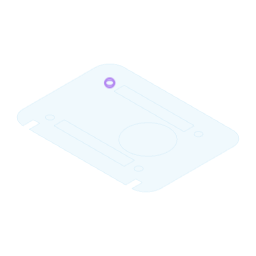
Seeed MT3620 Mini Dev Case (Autodesk Fusion 360 design; units mm, degrees)
Autodesk Fusion 360 part; units mm, degrees
sketch "Sketch1" plane through (0, 0, 0) normal (0, 1, 0) x (1, 0, 0)
  circle A0 centre (8.5, -10) radius 1.575
  circle A1 centre (51.5, -10) radius 1.575
  circle A2 centre (8.5, -39) radius 1.575
  circle A3 centre (51.5, -39) radius 1.575
  line L0 (5.5, 0) -> (58.2, 0)
  line L1 (65.2, -7) -> (65.2, -42)
  line L2 (58.2, -49) -> (5.5, -49)
  line L3 (-1.5, -42) -> (-1.5, -7)
  arc A4 (5.5, 0) -> (-1.5, -7) centre (5.5, -7) ccw
  arc A5 (65.2, -7) -> (58.2, 0) centre (58.2, -7) ccw
  arc A6 (-1.5, -42) -> (5.5, -49) centre (5.5, -42) ccw
  arc A7 (58.2, -49) -> (65.2, -42) centre (58.2, -42) ccw
  circle A8 centre (9, -34) radius 1
  line L4 (29.5, -28.775) -> (32, -28.775) construction
  line L5 (32, -28.775) -> (32, -35.275) construction
  line L6 (32, -35.275) -> (29.5, -35.275) construction
  line L7 (29.5, -35.275) -> (29.5, -28.775) construction
  circle A9 centre (8.5, -39) radius 2.075 construction
  circle A10 centre (8.5, -10) radius 2.075 construction
  circle A11 centre (51.5, -10) radius 2.075 construction
  circle A12 centre (51.5, -39) radius 2.075 construction
  line L8 (33, -27.775) -> (33, -36.275)
  line L9 (33, -36.275) -> (28.5, -36.275)
  line L10 (28.5, -36.275) -> (28.5, -27.775)
  line L11 (28.5, -27.775) -> (33, -27.775)
  line L12 (12.8, -11.5462) -> (11.2, -11.5462) construction
  line L13 (11.2, -11.5462) -> (11.2, -13.4538) construction
  line L14 (11.2, -13.4538) -> (12.8, -13.4538) construction
  line L15 (12.8, -13.4538) -> (12.8, -11.5462) construction
  line L16 (12.8, -11.5462) -> (11.2, -13.4538) construction
  line L17 (11.2, -11.5462) -> (12.8, -13.4538) construction
  line L18 (12.8, -9.2336) -> (11.2, -9.2336) construction
  line L19 (11.2, -9.2336) -> (11.2, -10.7664) construction
  line L20 (11.2, -10.7664) -> (12.8, -10.7664) construction
  line L21 (12.8, -10.7664) -> (12.8, -9.2336) construction
  line L22 (12.8, -9.2336) -> (11.2, -10.7664) construction
  line L23 (11.2, -9.2336) -> (12.8, -10.7664) construction
  line L24 (11.2, -9.2336) -> (11.2, -13.4538)
  line L25 (11.2, -13.4538) -> (12.8, -13.4538)
  line L26 (12.8, -13.4538) -> (12.8, -9.2336)
  line L27 (12.8, -9.2336) -> (11.2, -9.2336)
  line L28 (8.5, -39) -> (51.5, -39) construction
  line L29 (51.5, -39) -> (51.5, -10) construction
  line L30 (51.5, -10) -> (8.5, -10) construction
  line L31 (8.5, -10) -> (8.5, -39) construction
  line L32 (14.3, -14.9538) -> (14.3, -7.7336)
  line L33 (14.3, -7.7336) -> (9.7, -7.7336)
  line L34 (9.7, -7.7336) -> (9.7, -14.9538)
  line L35 (9.7, -14.9538) -> (14.3, -14.9538)
  point P0 (12, -10)
  point P1 (12, -12.5)
  point P2 (12, -12.5)
  point P3 (12, -10)
  dimension "d1" = 3.15
  dimension "d2" = 3.15
  dimension "d3" = 3.15
  dimension "d4" = 3.15
  dimension "d13" = 7
  dimension "d14" = 7
  dimension "d15" = 7
  dimension "d16" = 7
  dimension "d17" = 2
  dimension "d18" = 5
  dimension "d19" = 0.5
  dimension "d21" = 23.5
  dimension "d22" = 2.5
  dimension "d23" = 6.5
  dimension "d24" = 4.15
  dimension "d25" = 4.15
  dimension "d26" = 4.15
  dimension "d27" = 4.15
  dimension "d29" = -1
  dimension "d30" = 3.5
  dimension "d39" = 29
  dimension "d40" = 29
  dimension "d41" = 10
  dimension "d42" = 10
  dimension "d50" = 43
  dimension "d88" = 1.5
  constraint horizontal L0
  constraint vertical L1
  constraint horizontal L2
  constraint vertical L3
  constraint tangent L3 A4
  constraint tangent L0 A4
  constraint tangent L0 A5
  constraint tangent L1 A5
  constraint tangent L3 A6
  constraint tangent L2 A6
  constraint tangent L2 A7
  constraint tangent L1 A7
  constraint horizontal L4
  constraint vertical L5
  constraint horizontal L6
  constraint vertical L7
  constraint concentric A2 A9
  constraint concentric A0 A10
  constraint concentric A1 A11
  constraint concentric A3 A12
  constraint horizontal L12
  constraint perpendicular L12 L13
  constraint parallel L12 L14
  constraint parallel L13 L15
  constraint coincident L16 P2
  constraint coincident L17 P2
  constraint coincident P2 P1
  constraint horizontal L18
  constraint perpendicular L18 L19
  constraint parallel L18 L20
  constraint parallel L19 L21
  constraint coincident L22 P3
  constraint coincident L23 P3
  constraint coincident P3 P0
  constraint perpendicular L14 L24
  constraint perpendicular L18 L26
  constraint horizontal L28
  constraint vertical L29
  constraint horizontal L30
  constraint vertical L31
  constraint coincident A1.centre A11.centre
  constraint coincident A2.centre A9.centre
  measures "d1" diameter of A0
  measures "d2" diameter of A1
  measures "d3" diameter of A2
  measures "d4" diameter of A3
  measures "d13" radius of A4
  measures "d14" radius of A5
  measures "d15" radius of A6
  measures "d16" radius of A7
  measures "d17" diameter of A8
  measures "d18" vertical distance of A2.centre A8.centre
  measures "d19" horizontal distance of A2.centre A8.centre
  measures "d21" distance of A2.centre L5
  measures "d22" distance of L4.start L4.end
  measures "d23" distance of L4.start L6.end
  measures "d24" diameter of A9
  measures "d25" diameter of A10
  measures "d26" diameter of A11
  measures "d27" diameter of A12
  measures "d30" distance of A0.centre P3
  measures "d39" distance of A1.centre A3.centre
  measures "d40" distance of A0.centre A2.centre
  measures "d41" distance of L2 L28
  measures "d42" distance of L0 L30
  measures "d50" distance of A0.centre A1.centre
extrude "Extrude1" add sketch "Sketch1" along normal blind 3 contours L0 L1 L2 L3 A4 A5 A6 A7 makes body 1
ref_plane "WorkPlane1" through (31.85, -10.5, 24.5) normal (0, -1, 0) x (-1, 0, 0)
sketch "Sketch2" plane through (31.85, -10.5, 21.35) normal (0, -1, 0) x (1, 0, 0)
  line L0 (-33.35, 20.65) -> (-33.35, -14.35)
  arc A0 (-26.35, 27.65) -> (-33.35, 20.65) centre (-26.35, 20.65) ccw
  line L1 (26.35, 27.65) -> (-26.35, 27.65)
  arc A1 (33.35, 20.65) -> (26.35, 27.65) centre (26.35, 20.65) ccw
  line L2 (33.35, -14.35) -> (33.35, 20.65)
  arc A2 (26.35, -21.35) -> (33.35, -14.35) centre (26.35, -14.35) ccw
  line L3 (-26.35, -21.35) -> (26.35, -21.35)
  arc A3 (-33.35, -14.35) -> (-26.35, -21.35) centre (-26.35, -14.35) ccw
  circle A4 centre (-23.35, 17.65) radius 1.575
  circle A5 centre (19.65, 17.65) radius 1.575
  circle A6 centre (19.65, -11.35) radius 1.575
  line L4 (19.65, 17.65) -> (19.65, 3.15) construction
  line L5 (19.65, 17.65) -> (19.65, -11.35) construction
  circle A7 centre (9.65, 3.15) radius 10
  line L6 (15.15, 20.15) -> (-18.85, 20.15)
  line L7 (-18.85, 20.15) -> (-18.85, 15.15)
  line L8 (-18.85, 15.15) -> (15.15, 15.15)
  line L9 (15.15, 15.15) -> (15.15, 20.15)
  line L10 (15.15, 20.15) -> (-18.85, 15.15) construction
  line L11 (-18.85, 20.15) -> (15.15, 15.15) construction
  line L12 (-23.35, 17.65) -> (19.65, 17.65) construction
  line L13 (-23.35, -11.35) -> (19.65, -11.35) construction
  line L14 (15.15, -8.85) -> (-18.85, -8.85)
  line L15 (-18.85, -8.85) -> (-18.85, -13.85)
  line L16 (-18.85, -13.85) -> (15.15, -13.85)
  line L17 (15.15, -13.85) -> (15.15, -8.85)
  line L18 (15.15, -8.85) -> (-18.85, -13.85) construction
  line L19 (-18.85, -8.85) -> (15.15, -13.85) construction
  arc A8 (-22.15, -10.3299) -> (-22.15, -12.3701) centre (-23.35, -11.35) ccw
  circle A9 centre (-23.35, -11.35) radius 1.575
  point P0 (-1.85, 17.65)
  point P1 (-1.85, -11.35)
  dimension "d37" = 14.5
  dimension "d38" = 29
  dimension "d43" = 20
  dimension "d44" = 34
  dimension "d45" = 5
  dimension "d46" = 34
  dimension "d47" = 5
  dimension "d89" = 3.15
  constraint coincident A5.centre L4.start
  constraint vertical L4
  constraint coincident A6.centre L5.end
  constraint coincident L4.end A7
  constraint horizontal L6
  constraint perpendicular L6 L7
  constraint parallel L6 L8
  constraint parallel L7 L9
  constraint coincident L10 P0
  constraint coincident L11 P0
  constraint coincident A4.centre L12.start
  constraint midpoint P0 L12
  constraint coincident L13.start A8.centre
  constraint horizontal L14
  constraint perpendicular L14 L15
  constraint parallel L14 L16
  constraint parallel L15 L17
  constraint coincident L18 P1
  constraint coincident L19 P1
  constraint midpoint L13 P1
  constraint concentric A8 A9
  measures "d37" distance of A5.centre L4.end
  measures "d38" distance of A5.centre A6.centre
  measures "d43" diameter of A7
  measures "d44" distance of L7.end L8.end
  measures "d45" distance of L6.end L7.end
  measures "d46" distance of L15.end L16.end
  measures "d47" distance of L14.end L15.end
  measures "d89" diameter of A9
extrude "Extrude2" add sketch "Sketch2" along normal blind 3 separate body makes body 2
sketch "Sketch3" plane through (0, 0, 0) normal (0, -1, 0) x (1, 0, 0)
  circle A0 centre (8.5, 39) radius 1.575
  circle A1 centre (51.5, 39) radius 1.575
  circle A2 centre (9, 34) radius 1
  line L0 (28.5, 27.775) -> (28.5, 36.275)
  line L1 (28.5, 36.275) -> (33, 36.275)
  line L2 (33, 36.275) -> (33, 27.775)
  line L3 (33, 27.775) -> (28.5, 27.775)
  circle A3 centre (51.5, 10) radius 1.575
  arc A4 (5.5, 49) -> (-1.5, 42) centre (5.5, 42) ccw
  line L4 (-1.5, 42) -> (-1.5, 7)
  arc A5 (-1.5, 7) -> (5.5, 0) centre (5.5, 7) ccw
  line L5 (5.5, 0) -> (58.2, 0)
  arc A6 (58.2, 0) -> (65.2, 7) centre (58.2, 7) ccw
  line L6 (65.2, 7) -> (65.2, 42)
  arc A7 (65.2, 42) -> (58.2, 49) centre (58.2, 42) ccw
  line L7 (58.2, 49) -> (5.5, 49)
  circle A8 centre (51.5, 10) radius 1.825
  circle A9 centre (51.5, 10) radius 1.25
  line L8 (9.7, 14.9538) -> (14.3, 14.9538)
  line L9 (14.3, 14.9538) -> (14.3, 7.7336)
  line L10 (14.3, 7.7336) -> (9.7, 7.7336)
  line L11 (9.7, 7.7336) -> (9.7, 8.9799)
  arc A10 (9.7, 11.0201) -> (9.7, 8.9799) centre (8.5, 10) ccw
  line L12 (9.7, 11.0201) -> (9.7, 14.9538)
  dimension "d52" = 3.65
  dimension "d53" = 2.5
  constraint concentric A3 A8
  constraint concentric A8 A9
  measures "d52" diameter of A8
  measures "d53" diameter of A9
extrude "Extrude3" add sketch "Sketch3" along normal blind 5 separate body contours A3 | A8 makes body 3
extrude "Extrude4" [suppressed]
sketch "Sketch4" plane through (0, 3, 0) normal (0, 1, 0) x (-1, 0, 0)
  circle A0 centre (-8.5, 39) radius 1.575
  circle A1 centre (-51.5, 39) radius 1.575
  circle A2 centre (-9, 34) radius 1
  line L0 (-28.5, 36.275) -> (-28.5, 27.775)
  line L1 (-28.5, 27.775) -> (-33, 27.775)
  line L2 (-33, 27.775) -> (-33, 36.275)
  line L3 (-33, 36.275) -> (-28.5, 36.275)
  circle A3 centre (-51.5, 10) radius 1.575
  arc A4 (1.5, 42) -> (-5.5, 49) centre (-5.5, 42) ccw
  line L4 (-5.5, 49) -> (-58.2, 49)
  arc A5 (-58.2, 49) -> (-65.2, 42) centre (-58.2, 42) ccw
  line L5 (-65.2, 42) -> (-65.2, 7)
  arc A6 (-65.2, 7) -> (-58.2, 0) centre (-58.2, 7) ccw
  line L6 (-58.2, 0) -> (-5.5, 0)
  arc A7 (-5.5, 0) -> (1.5, 7) centre (-5.5, 7) ccw
  line L7 (1.5, 7) -> (1.5, 42)
  line L8 (-5.5, 49) -> (-8.5, 49)
  line L9 (-8.5, 49) -> (-8.5, 44)
  line L10 (-8.5, 44) -> (-5.5, 44)
  line L11 (-5.5, 44) -> (-5.5, 49)
  line L12 (-58.2, 49) -> (-55.2, 49)
  line L13 (-55.2, 49) -> (-55.2, 44)
  line L14 (-55.2, 44) -> (-58.2, 44)
  line L15 (-58.2, 44) -> (-58.2, 49)
  line L16 (-14.3, 14.9538) -> (-9.7, 14.9538)
  line L17 (-9.7, 14.9538) -> (-9.7, 11.0201)
  arc A8 (-9.7, 8.9799) -> (-9.7, 11.0201) centre (-8.5, 10) ccw
  line L18 (-9.7, 8.9799) -> (-9.7, 7.7336)
  line L19 (-9.7, 7.7336) -> (-14.3, 7.7336)
  line L20 (-14.3, 7.7336) -> (-14.3, 14.9538)
  dimension "d59" = 3
  dimension "d60" = 5
  dimension "d61" = 3
  dimension "d62" = 5
  constraint horizontal L8
  constraint vertical L9
  constraint horizontal L10
  constraint vertical L11
  constraint coincident A4.end L4.start
  constraint horizontal L12
  constraint vertical L13
  constraint horizontal L14
  constraint vertical L15
  constraint coincident L4.end A5.start
  measures "d59" distance of A4.end L8.end
  measures "d60" distance of A4.end L10.end
  measures "d61" distance of L4.end L12.end
  measures "d62" distance of L4.end L14.end
extrude "Extrude5" cut sketch "Sketch4" against normal blind 20 contours L4 L8 L9 L10 L11 | L4 L12 L13 L14 L15 bodies 1 2
ref_plane "WorkPlane2" through (55.2, 1.5, 46.5) normal (1, 0, 0) x (0, 0, 1)
sketch "Sketch6" plane through (55.2, 1.5, 46.5) normal (1, 0, 0) x (0, 0, -1)
  line L0 (4.5, -12) -> (4.5, -1.5) construction
  line L1 (-11.5, 5.7574) -> (-11.5, -41.7574)
  line L2 (-3, -40.5147) -> (-3, 4.5147)
  line L3 (-4.7574, 8.7574) -> (-19.8241, 23.8241)
  line L4 (-3, 7) -> (22, 7) construction
  line L5 (-20.6777, 23.4706) -> (-20.6777, 17.0061)
  line L6 (-20.0919, 15.5919) -> (-12.3787, 7.8787)
  line L7 (-4.7574, -44.7574) -> (-19.8241, -59.8241)
  line L8 (-3, -43) -> (22, -43) construction
  line L9 (-20.6777, -59.4706) -> (-20.6777, -53.0061)
  line L10 (-20.0919, -51.5919) -> (-12.3787, -43.8787)
  arc A0 (-19.8241, 23.8241) -> (-20.6777, 23.4706) centre (-20.1777, 23.4706) ccw
  arc A1 (-20.6777, -59.4706) -> (-19.8241, -59.8241) centre (-20.1777, -59.4706) ccw
  arc A2 (-20.0919, -51.5919) -> (-20.6777, -53.0061) centre (-18.6777, -53.0061) ccw
  arc A3 (-20.6777, 17.0061) -> (-20.0919, 15.5919) centre (-18.6777, 17.0061) ccw
  arc A4 (-3, 4.5147) -> (-4.7574, 8.7574) centre (-9, 4.5147) ccw
  arc A5 (-4.7574, -44.7574) -> (-3, -40.5147) centre (-9, -40.5147) ccw
  arc A6 (-12.3787, -43.8787) -> (-11.5, -41.7574) centre (-14.5, -41.7574) ccw
  arc A7 (-11.5, 5.7574) -> (-12.3787, 7.8787) centre (-14.5, 5.7574) ccw
  point P0 (-11.5, 7)
  point P1 (-20.6777, 24.6777)
  point P2 (-20.6777, 16.1777)
  point P3 (-20.6777, -60.6777)
  point P4 (-20.6777, -52.1777)
  dimension "d69" = 8.5
  dimension "d70" = 50
  dimension "d71" = 135
  dimension "d72" = 25
  dimension "d74" = 8.5
  dimension "d75" = 135
  dimension "d76" = 25
  dimension "d77" = 8.5
  dimension "d78" = 0.5
  dimension "d79" = 0.5
  dimension "d80" = 2
  dimension "d81" = 2
  dimension "d82" = 6
  dimension "d83" = 6
  dimension "d84" = 3
  dimension "d85" = 3
  constraint vertical L0
  constraint vertical L1
  constraint vertical L2
  constraint horizontal L4
  constraint vertical L5
  constraint horizontal L8
  constraint parallel L1 L9
  constraint coincident P1 L5
  constraint coincident P1 L3
  constraint tangent L5 A0
  constraint tangent L3 A0
  constraint coincident P3 L9
  constraint coincident P3 L7
  constraint tangent L9 A1
  constraint tangent L7 A1
  constraint coincident P4 L9
  constraint coincident P4 L10
  constraint tangent L9 A2
  constraint tangent L10 A2
  constraint coincident P2 L5
  constraint coincident P2 L6
  constraint tangent L5 A3
  constraint tangent L6 A3
  constraint coincident L4.start L3
  constraint coincident L4.start L2
  constraint tangent L3 A4
  constraint tangent L2 A4
  constraint coincident L8.start L2
  constraint coincident L8.start L7
  constraint tangent L2 A5
  constraint tangent L7 A5
  constraint tangent L10 A6
  constraint tangent L1 A6
  constraint coincident P0 L6
  constraint coincident P0 L1
  constraint tangent L6 A7
  constraint tangent L1 A7
  measures "d69" distance of L4.start P0
  measures "d70" distance of L4.start L8.start
  measures "d71" angle of L3 L4
  measures "d72" distance of L4.start P1
  measures "d74" distance of P1 P2
  measures "d75" angle of L7 L8
  measures "d76" distance of L8.start P3
  measures "d77" distance of P3 P4
  measures "d78" radius of A0
  measures "d79" radius of A1
  measures "d80" radius of A2
  measures "d81" radius of A3
  measures "d82" radius of A4
  measures "d83" radius of A5
  measures "d84" radius of A6
  measures "d85" radius of A7
extrude "Extrude6" add sketch "Sketch6" along normal blind 3 separate body makes body 4
sketch "Side 1 For Lasercut" plane through (0, 3, 0) normal (0, 1, 0) x (-1, 0, 0)
  line L0 (-8.5, 44) -> (-8.5, 49)
  line L1 (-8.5, 49) -> (-55.2, 49)
  line L2 (-55.2, 49) -> (-55.2, 44)
  line L3 (-55.2, 44) -> (-58.2, 44)
  line L4 (-58.2, 44) -> (-58.2, 49)
  arc A0 (-58.2, 49) -> (-65.2, 42) centre (-58.2, 42) ccw
  line L5 (-65.2, 42) -> (-65.2, 7)
  arc A1 (-65.2, 7) -> (-58.2, 0) centre (-58.2, 7) ccw
  line L6 (-58.2, 0) -> (-5.5, 0)
  arc A2 (-5.5, 0) -> (1.5, 7) centre (-5.5, 7) ccw
  line L7 (1.5, 7) -> (1.5, 42)
  arc A3 (1.5, 42) -> (-5.5, 49) centre (-5.5, 42) ccw
  line L8 (-5.5, 49) -> (-5.5, 44)
  line L9 (-5.5, 44) -> (-8.5, 44)
  circle A4 centre (-8.5, 39) radius 1.575
  circle A5 centre (-51.5, 39) radius 1.575
  circle A6 centre (-9, 34) radius 1
  line L10 (-28.5, 36.275) -> (-28.5, 27.775)
  line L11 (-28.5, 27.775) -> (-33, 27.775)
  line L12 (-33, 27.775) -> (-33, 36.275)
  line L13 (-33, 36.275) -> (-28.5, 36.275)
  circle A7 centre (-51.5, 10) radius 1.575
  line L14 (-14.3, 14.9538) -> (-9.7, 14.9538)
  line L15 (-9.7, 14.9538) -> (-9.7, 11.0201)
  arc A8 (-9.7, 8.9799) -> (-9.7, 11.0201) centre (-8.5, 10) ccw
  line L16 (-9.7, 8.9799) -> (-9.7, 7.7336)
  line L17 (-9.7, 7.7336) -> (-14.3, 7.7336)
  line L18 (-14.3, 7.7336) -> (-14.3, 14.9538)
sketch "Side 2 For Lasercut" plane through (0, -13.5, 0) normal (0, -1, 0) x (1, 0, 0)
  circle A0 centre (41.5, 24.5) radius 10
  circle A1 centre (51.5, 10) radius 1.575
  circle A2 centre (51.5, 39) radius 1.575
  circle A3 centre (8.5, 39) radius 1.575
  line L0 (47, 41.5) -> (47, 36.5)
  line L1 (47, 36.5) -> (13, 36.5)
  line L2 (13, 36.5) -> (13, 41.5)
  line L3 (13, 41.5) -> (47, 41.5)
  line L4 (47, 12.5) -> (47, 7.5)
  line L5 (47, 7.5) -> (13, 7.5)
  line L6 (13, 7.5) -> (13, 12.5)
  line L7 (13, 12.5) -> (47, 12.5)
  line L8 (8.5, 49) -> (8.5, 44)
  line L9 (8.5, 44) -> (5.5, 44)
  line L10 (5.5, 44) -> (5.5, 49)
  arc A4 (5.5, 49) -> (-1.5, 42) centre (5.5, 42) ccw
  line L11 (-1.5, 42) -> (-1.5, 7)
  arc A5 (-1.5, 7) -> (5.5, 0) centre (5.5, 7) ccw
  line L12 (5.5, 0) -> (58.2, 0)
  arc A6 (58.2, 0) -> (65.2, 7) centre (58.2, 7) ccw
  line L13 (65.2, 7) -> (65.2, 42)
  arc A7 (65.2, 42) -> (58.2, 49) centre (58.2, 42) ccw
  line L14 (58.2, 49) -> (58.2, 44)
  line L15 (58.2, 44) -> (55.2, 44)
  line L16 (55.2, 44) -> (55.2, 49)
  line L17 (55.2, 49) -> (8.5, 49)
  circle A8 centre (8.5, 10) radius 1.575
sketch "Stand For Lasercut" plane through (58.2, 0, 0) normal (1, 0, 0) x (0, 0, -1)
  arc A0 (-66.5919, -50.0919) -> (-67.1777, -51.5061) centre (-65.1777, -51.5061) ccw
  line L0 (-67.1777, -51.5061) -> (-67.1777, -57.9706)
  arc A1 (-67.1777, -57.9706) -> (-66.3241, -58.3241) centre (-66.6777, -57.9706) ccw
  line L1 (-66.3241, -58.3241) -> (-51.2574, -43.2574)
  arc A2 (-51.2574, -43.2574) -> (-49.5, -39.0147) centre (-55.5, -39.0147) ccw
  line L2 (-49.5, -39.0147) -> (-49.5, 6.0147)
  arc A3 (-49.5, 6.0147) -> (-51.2574, 10.2574) centre (-55.5, 6.0147) ccw
  line L3 (-51.2574, 10.2574) -> (-66.3241, 25.3241)
  arc A4 (-66.3241, 25.3241) -> (-67.1777, 24.9706) centre (-66.6777, 24.9706) ccw
  line L4 (-67.1777, 24.9706) -> (-67.1777, 18.5061)
  arc A5 (-67.1777, 18.5061) -> (-66.5919, 17.0919) centre (-65.1777, 18.5061) ccw
  line L5 (-66.5919, 17.0919) -> (-58.8787, 9.3787)
  arc A6 (-58, 7.2574) -> (-58.8787, 9.3787) centre (-61, 7.2574) ccw
  line L6 (-58, 7.2574) -> (-58, -40.2574)
  arc A7 (-58.8787, -42.3787) -> (-58, -40.2574) centre (-61, -40.2574) ccw
  line L7 (-58.8787, -42.3787) -> (-66.5919, -50.0919)
hidden bodies 1 2 3 4
equation "d50 = 39.85 mm + 3.15 mm"
equation "d71 = 180 deg - 45 deg"
named bodies: "Side 1", "Side 2", "Standoff", "Stand"
